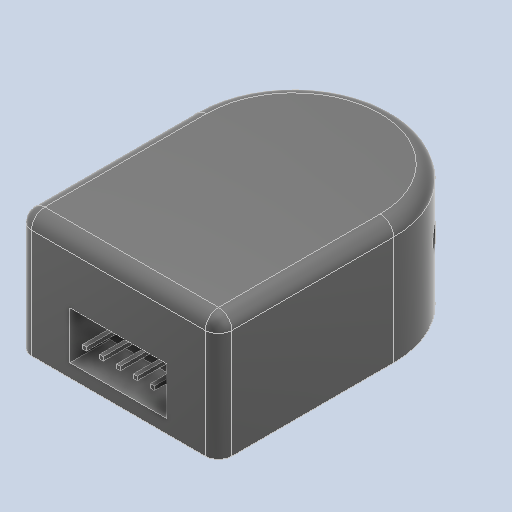
# Autodesk Inventor part: HEDM-5500_13_V1
Saved by Autodesk Inventor 2023 (Build 270158000, 158)
## iProperties
Created: 2023-02-13
Part Number: HEDM-5500_13_V1
Material: ABS-Kunststoff
Document SubType Name: Modeling
Designer: Mathi
Density: 1.06 g/cm^3
Appearance: Glatt - Weiß
Author: Mathi
Autodesk Inventor part; units mm, degrees
ref_plane "YZ Plane" through (0, 0, 0) normal (1, 0, 0) x (0, 1, 0)
ref_plane "XY Plane" through (0, 0, 0) normal (0, 0, 1) x (1, 0, 0)
sketch "Skizze1" plane through (0, 0, 0) normal (0, 1, 0) x (-1, 0, 0)
  circle A0 centre (0, 0) radius 4
  arc A1 (-15, 0) -> (15, 0) centre (0, 0) ccw
  line L0 (15, 0) -> (15, 26.2)
  line L1 (15, 26.2) -> (-15, 26.2)
  line L2 (-15, 26.2) -> (-15, 0)
  circle A2 centre (0, 0) radius 10.45 construction
  circle A3 centre (0, -10.45) radius 0.8
  circle A4 centre (9.05, 5.225) radius 0.8
  circle A5 centre (-9.05, 5.225) radius 0.8
  circle A6 centre (0, 0) radius 9.525 construction
  circle A7 centre (9.525, 0) radius 1.25
  circle A8 centre (-9.525, 0) radius 1.25
  line L3 (9.525, 0) -> (-9.525, 0) construction
  line L4 (9.05, 5.225) -> (-9.05, 5.225) construction
  line L5 (0, -10.45) -> (-9.05, 5.225) construction
  line L6 (0, -10.45) -> (9.05, 5.225) construction
  line L7 (0, 0) -> (0, -10.45) construction
  line L8 (0, 0) -> (-11.4907, -9.6418)
  line L9 (-11.4907, -9.6418) -> (-2.8406, -2.3835)
  line L10 (-2.8406, -2.3835) -> (-3.8048, -1.2345)
  line L11 (-3.8048, -1.2345) -> (-12.4548, -8.4927)
  line L12 (-12.4548, -8.4927) -> (-11.4907, -9.6418)
  dimension "d1" = 8
  dimension "d0" = 30
  dimension "d2" = 26.2
  dimension "d3" = 20.9
  dimension "d4" = 1.6
  dimension "d5" = 19.05
  dimension "d6" = 2.5
  dimension "d12" = 3
  dimension "d13" = 40
  constraints: 26 end point, 8 centre point, 8 point on circle, 4 coincident, 3 equal length, 3 equal radius, 3 vertical, 2 parallel, 2 perpendicular, 2 tangent, 1 horizontal, 1 midpoint, 1 point on line, 3 other
  measures "d0" diameter of A1
  measures "d2" distance from line of A1.centre L1
  measures "d3" diameter of A2
  measures "d4" diameter of A3
  measures "d5" diameter of A6
  measures "d6" diameter of A7
  measures "d12" diameter of L11 L8
  measures "d13" angle of L8 L3
extrude "Extrusion1" add sketch "Skizze1" along normal blind 18.3 contours A0 L11 A1 L2 L1 L0 L8 | A0 L8 A1 L11
sketch "Skizze2" plane through (0, 18.3, 0) normal (0, 1, 0) x (1, 0, 0)
  circle A0 centre (0, 10.45) radius 0.8 projected
  circle A1 centre (-9.525, 0) radius 1.25 projected
  circle A2 centre (-9.05, -5.225) radius 0.8 projected
  circle A3 centre (0, 0) radius 4 projected
  circle A4 centre (9.05, -5.225) radius 0.8 projected
  circle A5 centre (9.525, 0) radius 1.25 projected
extrude "Extrusion2" add sketch "Skizze2" against normal blind 1
fillet "Rundung1" radius 2 6 edges at (0, 18.3, -15) (15, 18.3, 13.1) (-15, 18.3, 13.1) (0, 18.3, 26.2) (-15, 9.15, 26.2) (15, 9.15, 26.2)
ref_plane "Arbeitsebene1" through (0, 9.9, 0) normal (0, 1, 0) x (-1, 0, 0)
sketch "Skizze3" plane through (0, 9.9, 0) normal (0, 1, 0) x (-1, 0, 0)
  line L0 (-3.8048, -1.2345) -> (-12.4548, -8.4927) projected
  line L1 (-2.8406, -2.3835) -> (-3.8048, -1.2345) projected
  line L2 (0, 0) -> (-11.4907, -9.6418) projected
  line L3 (-12.4548, -8.4927) -> (-11.4907, -9.6418) projected
  line L4 (-2.8406, -2.3835) -> (-11.4907, -9.6418)
  constraints: 2 end point
revolve "Umdrehung1" cut sketch "Skizze3" angle 360 about axis through (0, 9.9, 0) along (0.7660444, 0, -0.6427876)
sketch "Skizze4" plane through (-13, 0, 26.2) normal (0, 0, 1) x (1, 0, 0)
  line L0 (0, 0) -> (26, 0) projected
  line L1 (5.75, 2) -> (20.25, 2)
  line L2 (20.25, 2) -> (20.25, 9.1)
  line L3 (20.25, 9.1) -> (5.75, 9.1)
  line L4 (5.75, 9.1) -> (5.75, 2)
  line L5 (13, 9.1) -> (13, 0) construction
  line L6 (12.7, 4.7) -> (13.3, 4.7)
  line L7 (13.3, 4.7) -> (13.3, 5.3)
  line L8 (13.3, 5.3) -> (12.7, 5.3)
  line L9 (12.7, 5.3) -> (12.7, 4.7)
  line L10 (12.7, 4.7) -> (13.3, 5.3) construction
  line L11 (13.3, 4.7) -> (12.7, 5.3) construction
  line L12 (15.84, 4.7) -> (15.84, 5.3)
  line L13 (15.84, 5.3) -> (15.24, 5.3)
  line L14 (15.24, 5.3) -> (15.24, 4.7)
  line L15 (15.24, 4.7) -> (15.84, 4.7)
  line L16 (18.38, 4.7) -> (18.38, 5.3)
  line L17 (18.38, 5.3) -> (17.78, 5.3)
  line L18 (17.78, 5.3) -> (17.78, 4.7)
  line L19 (17.78, 4.7) -> (18.38, 4.7)
  line L20 (10.76, 4.7) -> (10.76, 5.3)
  line L21 (10.76, 5.3) -> (10.16, 5.3)
  line L22 (10.16, 5.3) -> (10.16, 4.7)
  line L23 (10.16, 4.7) -> (10.76, 4.7)
  line L24 (13.3, 4.7) -> (13.3, 5.3)
  line L25 (13.3, 5.3) -> (12.7, 5.3)
  line L26 (12.7, 5.3) -> (12.7, 4.7)
  line L27 (12.7, 4.7) -> (13.3, 4.7)
  line L28 (15.84, 4.7) -> (15.84, 5.3)
  line L29 (15.84, 5.3) -> (15.24, 5.3)
  line L30 (15.24, 5.3) -> (15.24, 4.7)
  line L31 (15.24, 4.7) -> (15.84, 4.7)
  line L32 (8.22, 4.7) -> (8.22, 5.3)
  line L33 (8.22, 5.3) -> (7.62, 5.3)
  line L34 (7.62, 5.3) -> (7.62, 4.7)
  line L35 (7.62, 4.7) -> (8.22, 4.7)
  line L36 (10.76, 4.7) -> (10.76, 5.3)
  line L37 (10.76, 5.3) -> (10.16, 5.3)
  line L38 (10.16, 5.3) -> (10.16, 4.7)
  line L39 (10.16, 4.7) -> (10.76, 4.7)
  line L40 (13.3, 4.7) -> (13.3, 5.3)
  line L41 (13.3, 5.3) -> (12.7, 5.3)
  line L42 (12.7, 5.3) -> (12.7, 4.7)
  line L43 (12.7, 4.7) -> (13.3, 4.7)
  point P0 (13, 5)
  dimension "d16" = 7.1
  dimension "d17" = 14.5
  dimension "d18" = 2
  dimension "d19" = 0.6
  dimension "d20" = 3
  dimension "d23" = 2.54
  dimension "d26" = 2.54
  constraints: 86 end point, 4 horizontal, 4 parallel, 3 midpoint, 3 perpendicular, 1 point on line, 1 vertical, 64 other
  measures "d16" distance of L3.end L1.start
  measures "d17" distance of L2.end L3.end
  measures "d18" distance between parallel lines of L1 L0
  measures "d19" distance of L8.end L7.end
  measures "d20" distance from line of point (13, 5) L1
  measures "d23" distance of L6.end L12.start
  measures "d26" distance of L6.end L20.start
extrude "Extrusion3" cut sketch "Skizze4" against normal blind 6
